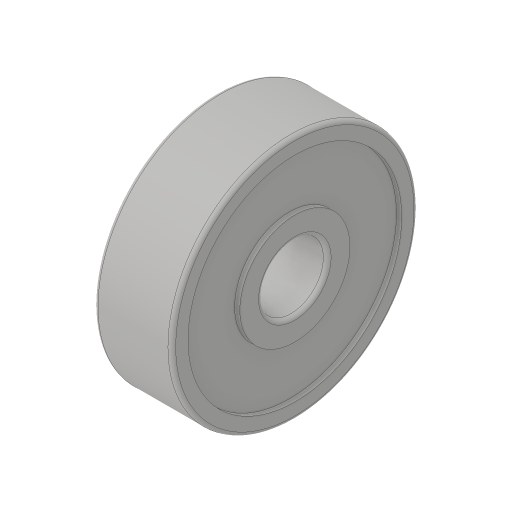
# Autodesk Inventor part: C-SE635ZZ
Saved by Autodesk Inventor 2024 (Build 280153000, 153)
## iProperties
Category: PARTsolutions
Company: MISUMI
Created: 2023-11-10
Part Number: C-SE635ZZ
Material: Generic
Catalog Web Link: www.cadenas.de
Description: C-SE___ZZ, C-SE___AZZ-Economy Stainless Miniature Deep Groove Ball Bearing - Double Shielded, Single Row
Vendor: MISUMI
Document SubType Name: Modeling
Designer: psAdmin
Manufacturer: MISUMI
Mass: 1.45529 g
Surface Area: 10.2334 cm^2
Volume: 1.45529 cm^3
Density: 1 g/cm^3
Appearance: PSOLRGB-175-175-175
PSOL_IDENT_0: {$CADENAS_DATA/23d-libs/misumi/metric/12_bearing_holders/c_se682zz.prj},174 {VTYP=3D},{NB=C-SE635ZZ}
PSOL_IDENT_1: ,{LINA=C-SE635ZZ},{NN=C-SE___ZZ, C-SE___AZZ},{DATE=29.05.2023 02:13:15},{GEOMDATE=25.05.2021 01:28:2
PSOL_IDENT_2: 4},{VERSION=},{LINEID=410},{WBVAR=},{WBNUMERIC=}  {NB=C-SE635ZZ},{LINA=C-SE635ZZ},{KT=DUMMY},{PN=C-S
PSOL_IDENT_3: E635ZZ},{TS=C-SE635ZZ},{DD=5.0},{D=19},{B=6.0},{RR=0.30},{A=5.2032},{BB=1.250},{C=1.750}
NB: C-SE635ZZ
NN: C-SE___ZZ, C-SE___AZZ
NT: Economy Stainless Miniature Deep Groove Ball Bearing - Double Shielded, Single Row
NBSYN: $PN.
LINA: C-SE635ZZ
CATALOG: Misumi
PN: C-SE635ZZ
TS: C-SE635ZZ
DD: 5
D: 19
B: 6
RR: 0.3
SUPPLIER: MISUMI
ARTICLENO: C-SE635ZZ
BOMINFO: C-SE635ZZ
CREATOR: CADENAS GmbH
Title: C-SE635ZZ
Author: Cadenas PARTsolutions
Comments: Economy Stainless Miniature Deep Groove Ball Bearing - Double Shielded, Single Row
Autodesk Inventor part; units mm, degrees
sketch "Sketch_1" plane through (0, 0, 0) normal (0, 0, 1) x (1, 0, 0)
  line L0 (5.7, 0) -> (0.3, 0)
  arc A0 (0, 2.8) -> (0.3, 2.5) centre (0.3, 2.8) ccw
  line L1 (0.3, 2.5) -> (5.7, 2.5)
  arc A1 (5.7, 2.5) -> (6, 2.8) centre (5.7, 2.8) ccw
  line L2 (6, 2.8) -> (6, 4.25)
  line L3 (6, 4.25) -> (5.6016, 4.25)
  line L4 (5.6016, 4.25) -> (5.6016, 8.25)
  line L5 (5.6016, 8.25) -> (6, 8.25)
  line L6 (6, 8.25) -> (6, 9.2)
  arc A2 (6, 9.2) -> (5.7, 9.5) centre (5.7, 9.2) ccw
  line L7 (5.7, 9.5) -> (0.3, 9.5)
  arc A3 (0.3, 9.5) -> (0, 9.2) centre (0.3, 9.2) ccw
  line L8 (0, 9.2) -> (0, 8.25)
  line L9 (0, 8.25) -> (0.3984, 8.25)
  line L10 (0.3984, 8.25) -> (0.3984, 4.25)
  line L11 (0.3984, 4.25) -> (0, 4.25)
  line L12 (0, 4.25) -> (0, 2.8)
  constraints: 26 end point, 8 point on circle, 4 centre point
revolve "Revolution1" add sketch "Sketch_1" angle 360 about axis through (5.7, 0, 0) along (1, 0, 0)
ref_plane "to_housing_XY" through (0, 0, 0) normal (1, 0, 0) x (0, 0, -1)
ref_plane "to_housing_YZ" through (0, 0, 0) normal (0, 0, -1) x (0, 1, 0)
ref_plane "to_housing_ZX" through (0, 0, 0) normal (0, 1, 0) x (1, 0, 0)
ref_plane "to_housing_center_XY" through (3, 0, 0) normal (1, 0, 0) x (0, 0, -1)
ref_plane "to_housing_center_YZ" through (3, 0, 0) normal (0, 0, -1) x (0, 1, 0)
ref_plane "to_housing_center_ZX" through (3, 0, 0) normal (0, 1, 0) x (1, 0, 0)
ref_plane "作業平面7" through (3, 0, 0) normal (1, 0, 0) x (0, 0, -1)
body "Solid1"
